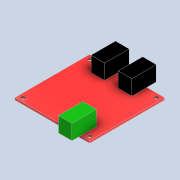
# Autodesk Inventor part: Drok L298 DC Motor Driver
Saved by Autodesk Inventor 2022 (Build 260153000, 153)
## iProperties
Created: 2022-01-02
Part Number: Drok L298 DC Motor Driver
Material: Generic
Document SubType Name: Modeling
Designer: Coy
Density: 1 g/cm^3
Appearance: Anodized - Black
Author: Coy
Autodesk Inventor part; units mm, degrees
ref_plane "YZ Plane" through (0, 0, 0) normal (1, 0, 0) x (0, 1, 0)
ref_plane "XZ Plane" through (0, 0, 0) normal (0, 1, 0) x (-1, 0, 0)
ref_plane "XY Plane" through (0, 0, 0) normal (0, 0, 1) x (1, 0, 0)
sketch "Sketch1" plane through (0, 0, 0) normal (0, 1, 0) x (-1, 0, 0)
  line L0 (0, 0) -> (55, 0)
  line L1 (55, 0) -> (55, 55)
  line L2 (55, 55) -> (0, 55)
  line L3 (0, 55) -> (0, 0)
  dimension "d0" = 55
  dimension "d1" = 55
  constraints: 8 end point, 2 parallel, 1 horizontal, 1 perpendicular
  measures "d0" distance of L2.end L1.end
  measures "d1" distance of L0.end L1.end
extrude "Extrusion1" add sketch "Sketch1" along normal blind 1.6
sketch "Sketch2" plane through (0, 1.6, 0) normal (0, 1, 0) x (1, 0, 0)
  line L0 (-52, -52) -> (-3, -52) construction
  line L1 (-3, -52) -> (-3, -3) construction
  line L2 (-3, -3) -> (-52, -3) construction
  line L3 (-52, -3) -> (-52, -52) construction
  line L4 (-52, -52) -> (-55, -52) construction
  line L5 (-55, 0) -> (-55, -55) construction
  line L6 (-52, -52) -> (-52, -55) construction
  line L7 (-55, -55) -> (0, -55) construction
  line L8 (-3, -3) -> (-3, 0) construction
  line L9 (0, 0) -> (-55, 0) construction
  line L10 (-3, -3) -> (0, -3) construction
  line L11 (0, -55) -> (0, 0) construction
  circle A0 centre (-52, -52) radius 1.5
  circle A1 centre (-52, -3) radius 1.5
  circle A2 centre (-3, -3) radius 1.5
  circle A3 centre (-3, -52) radius 1.5
  dimension "d4" = 49
  dimension "d5" = 49
  dimension "d6" = 3
  dimension "d7" = 3
  dimension "d8" = 3
  dimension "d9" = 3
  constraints: 16 end point, 4 centre point, 4 coincident, 4 parallel, 4 point on line, 3 perpendicular, 2 vertical, 1 horizontal
  measures "d4" distance of L2.end L1.end
  measures "d5" distance of L1.end L0.end
  measures "d6" diameter of A0
  measures "d7" diameter of A1
  measures "d8" diameter of A2
  measures "d9" diameter of A3
extrude "Extrusion2" cut sketch "Sketch2" against normal up to next
sketch "Sketch3" plane through (0, 1.6, 0) normal (0, 1, 0) x (1, 0, 0)
  line L0 (-6.5, -43.5) -> (-16.5, -43.5)
  line L1 (-16.5, -43.5) -> (-16.5, -61.5)
  line L2 (-16.5, -61.5) -> (-6.5, -61.5)
  line L3 (-6.5, -61.5) -> (-6.5, -43.5)
  line L4 (-55, -55) -> (0, -55) projected
  point P0 (0, 0)
  dimension "d12" = 10
  dimension "d13" = 18
  dimension "d14" = 6.5
  dimension "d15" = 6.5
  constraints: 8 end point, 2 parallel, 1 horizontal, 1 perpendicular
  measures "d12" distance of L2.end L1.end
  measures "d13" distance of L1.end L0.end
  measures "d14" distance between parallel lines of L4 L2
  measures "d15" distance from line of L4.end L3
extrude "Extrusion3" add sketch "Sketch3" along normal blind 11
sketch "Sketch4" plane through (0, 1.6, 0) normal (0, 1, 0) x (1, 0, 0)
  line L0 (-13, -11) -> (-23, -11)
  line L1 (-23, -11) -> (-23, 7)
  line L2 (-23, 7) -> (-13, 7)
  line L3 (-13, 7) -> (-13, -11)
  line L4 (-33, -11) -> (-43, -11)
  line L5 (-43, -11) -> (-43, 7)
  line L6 (-43, 7) -> (-33, 7)
  line L7 (-33, 7) -> (-33, -11)
  line L8 (0, -55) -> (0, 0) projected
  line L9 (0, 0) -> (-55, 0) projected
  dimension "d18" = 10
  dimension "d19" = 10
  dimension "d20" = 18
  dimension "d21" = 18
  dimension "d22" = 10
  dimension "d23" = 13
  dimension "d24" = 7
  constraints: 16 end point, 4 parallel, 2 horizontal, 2 perpendicular, 1 point on line
  measures "d18" distance of L5.end L6.end
  measures "d19" distance of L1.end L2.end
  measures "d20" distance of L4.end L5.end
  measures "d21" distance of L0.end L1.end
  measures "d22" distance between parallel lines of L1 L7
  measures "d23" distance between parallel lines of L8 L3
  measures "d24" distance between parallel lines of L9 L2
extrude "Extrusion4" add sketch "Sketch4" along normal blind 11
equation "\"d1\" = d0"
equation "\"d7\" = d6"
equation "\"d8\" = d6"
equation "\"d9\" = d6"
equation "\"d10\" = d5"
equation "\"d19\" = d18"
equation "\"d21\" = d20"
body "Solid1"
